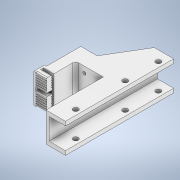
# Autodesk Inventor part: Soporte Linear Rail X
Saved by Autodesk Inventor 2021 (Build 250183000, 183)
## iProperties
Created: 2023-01-21
Part Number: Soporte Linear Rail X
Material: Plástico ABS
Document SubType Name: Modeling
Designer: Diego.labarca
Density: 1.06 g/cm^3
Appearance: Suave - Blanco
Author: Diego.labarca
Autodesk Inventor part; units mm, degrees
ref_plane "YZ Plane" through (0, 0, 0) normal (1, 0, 0) x (0, 1, 0)
ref_plane "XZ Plane" through (0, 0, 0) normal (0, 1, 0) x (-1, 0, 0)
ref_plane "XY Plane" through (0, 0, 0) normal (0, 0, 1) x (1, 0, 0)
sketch "Boceto1" plane through (0, 0, 0) normal (0, 0, 1) x (1, 0, 0)
  line L0 (-10, 11) -> (10, 11)
  line L1 (10, 11) -> (10, -11)
  line L2 (10, -11) -> (-10, -11)
  line L3 (-10, -11) -> (-10, 11)
  line L4 (1.6972, 0) -> (0, 0)
  line L5 (0, 0) -> (0, 1.3941)
  dimension "d11" = 22
  dimension "d12" = 20
  constraints: 12 end point, 2 horizontal, 2 parallel, 2 perpendicular, 2 other
  measures "d11" distance of L0.end L1.end
  measures "d12" distance of L0.start L0.end
extrude "Extrusión1" add sketch "Boceto1" along normal blind 15
sketch "Boceto5" plane through (0, 0, 15) normal (0, 0, 1) x (1, 0, 0)
  line L0 (-10, -11) -> (10, -11) projected
  line L1 (-10, -11) -> (35, -11)
  line L2 (35, -11) -> (35, -15)
  line L3 (35, -15) -> (-10, -15)
  line L4 (-10, -15) -> (-10, -11)
  line L5 (10, -11) -> (10, 11) projected
  line L6 (-10, 11) -> (-10, -11) projected
  line L7 (-10, 10) -> (35, 10)
  line L8 (35, 10) -> (35, 14)
  line L9 (35, 14) -> (-10, 14)
  line L10 (-10, 14) -> (-10, 10)
  line L11 (10, 11) -> (-10, 11) projected
  point P0 (0, 0)
  point P1 (10, 10)
  dimension "d25" = 4
  dimension "d26" = 25
  dimension "d28" = 4
  dimension "d29" = 1
  constraints: 16 end point, 4 parallel, 2 horizontal, 2 perpendicular, 1 collinear, 1 point on line
  measures "d25" distance of L1.end L2.end
  measures "d26" distance between parallel lines of L5 L2
  measures "d28" distance of L8.end L7.end
  measures "d29" distance from line of L7.start L11
extrude "Extrusión5" add sketch "Boceto5" against normal up to surface (15 mm away) contours L0 L1 L2 L3 L4 | L5 L11 L10 L9 L8 L7
sketch "Boceto7" plane through (0, 0, 0) normal (0, 0, -1) x (-1, 0, 0)
  line L0 (10, 14) -> (-35, 14) projected
  line L1 (-35, 10) -> (-10, 10) projected
  line L2 (-35, 14) -> (-15, 14)
  line L3 (-15, 14) -> (-15, 10)
  line L4 (-15, 10) -> (-35, 10)
  line L5 (-35, 10) -> (-35, 14)
  line L6 (-10, -11) -> (-35, -11) projected
  line L7 (-35, -15) -> (10, -15) projected
  line L8 (-35, -11) -> (-15, -11)
  line L9 (-15, -11) -> (-15, -15)
  line L10 (-15, -15) -> (-35, -15)
  line L11 (-35, -15) -> (-35, -11)
  point P0 (0, 0)
  point P1 (-15, 14)
  dimension "d32" = 20
  constraints: 16 end point, 4 parallel, 3 point on line, 2 horizontal, 2 perpendicular
  measures "d32" distance of L3.end L4.end
extrude "Extrusión6" add sketch "Boceto7" along normal blind 35 and the other way blind 71
ref_plane "Plano de trabajo1" through (0, 0, 7.5) normal (0, 0, -1) x (-1, 0, 0)
sketch "Boceto10" plane through (0, 0, -35) normal (0, 0, -1) x (-1, 0, 0)
  line L0 (10, 14) -> (-15, 14) projected
  line L1 (-10, 10) -> (-15, 10) projected
  line L2 (-15, 14) -> (-14, 14)
  line L3 (-14, 14) -> (-14, 10)
  line L4 (-14, 10) -> (-15, 10)
  line L5 (-15, 10) -> (-15, 14)
  line L6 (-15, -15) -> (-15, -11) projected
  line L7 (10, -15) -> (-15, -15) projected
  line L8 (-15, -11) -> (-14, -11)
  line L9 (-14, -11) -> (-14, -15)
  line L10 (-14, -15) -> (-15, -15)
  line L11 (-15, -15) -> (-15, -11)
  line L12 (-14, -15) -> (-11, -15)
  line L13 (-11, -15) -> (-11, 14)
  line L14 (-11, 14) -> (-14, 14)
  line L15 (-14, 14) -> (-14, -15)
  point P0 (0, 0)
  point P1 (-11, -15)
  point P2 (-11, 10)
  point P3 (-11, 14)
  dimension "d60" = 1
  dimension "d61" = 1
  dimension "d62" = 3
  constraints: 24 end point, 6 parallel, 3 horizontal, 3 perpendicular, 3 point on line
  measures "d60" distance of L3.end L4.end
  measures "d61" distance of L9.end L10.end
  measures "d62" distance of L14.end L13.end
extrude "Extrusión9" add sketch "Boceto10" against normal up to surface (106 mm away)
sketch "Boceto11" plane through (-10, 14, 15) normal (0, 1, 0) x (1, 0, 0)
  line L0 (0, 0) -> (0, 15) projected
  circle A0 centre (35, 7.5) radius 2.5
  circle A1 centre (35, 40) radius 2.5
  circle A2 centre (35, -41) radius 2.5
  line L1 (21, 50) -> (45, 50) projected
  line L2 (45, -56) -> (21, -56) projected
  line L3 (45, -56) -> (45, 50) projected
  point P0 (10, 15)
  dimension "d65" = 5
  dimension "d66" = 5
  dimension "d67" = 5
  dimension "d69" = 10
  dimension "d70" = 15
  dimension "d73" = 10
  dimension "d74" = 10
  dimension "d75" = 10
  constraints: 3 centre point
  measures "d65" diameter of A0
  measures "d66" diameter of A2
  measures "d67" diameter of A1
  measures "d69" distance from line of A1.centre L1
  measures "d70" distance from line of L2 A2.centre
  measures "d73" distance from line of L3 A2.centre
  measures "d74" distance from line of L3 A0.centre
  measures "d75" distance from line of L3 A1.centre
extrude "Extrusión10" cut sketch "Boceto11" against normal up to surface (29 mm away)
sketch "Boceto13" plane through (0, 0, 0) normal (0, 0, -1) x (-1, 0, 0)
  line L0 (-10, -11) -> (-10, 10) projected
  line L1 (-11, 10) -> (-10, 10) projected
  line L2 (-10, -11) -> (-11, -11) projected
  line L3 (-11, -15) -> (-11, 14) projected
  point P0 (0, 0)
extrude "Extrusión12" add sketch "Boceto13" against normal up to surface (15 mm away)
sketch "Boceto14" plane through (-10, 14, 15) normal (0, 1, 0) x (1, 0, 0)
  line L0 (21, 50) -> (45, 50) projected
  line L1 (0, 15) -> (21, 50)
  line L2 (21, 50) -> (21, 15) projected
  line L3 (0, 15) -> (21, 15) projected
  point P0 (10, 15)
  constraints: 2 end point
extrude "Extrusión13" add sketch "Boceto14" against normal up to surface (29 mm away)
sketch "Boceto12" plane through (11, -15, -35) normal (-1, 0, 0) x (0, 0, 1)
  circle A0 centre (15, 15) radius 2.5
  line L0 (0, 29) -> (35, 29) projected
  line L1 (0, 0) -> (0, 29) projected
  circle A1 centre (80, 15) radius 2.5
  line L2 (50, 29) -> (106, 29) projected
  line L3 (50, 29) -> (50, 0) projected
  line L4 (106, 0) -> (106, 29) projected
  point P0 (35, 15)
  dimension "d76" = 5
  dimension "d77" = 14
  dimension "d78" = 15
  dimension "d79" = 5
  dimension "d80" = 14
  dimension "d84" = 26
  constraints: 2 centre point
  measures "d76" diameter of A0
  measures "d77" distance from line of L0 A0.centre
  measures "d78" distance from line of L1 A0.centre
  measures "d79" diameter of A1
  measures "d80" distance from line of A1.centre L2
  measures "d84" distance from line of L4 A1.centre
extrude "Extrusión11" cut sketch "Boceto12" against normal through all both and the other way through all
sketch "Boceto15" plane through (-10, -15, 15) normal (-1, 0, 0) x (0, 0, 1)
  circle A0 centre (-35, 15) radius 2.5 projected
  circle A1 centre (-35, 15) radius 2.5 projected
  circle A2 centre (-35, 15) radius 5
  point P0 (-15, 15)
  dimension "d90" = 10
  constraints: 1 centre point, 1 coincident
  measures "d90" diameter of A2
extrude "Extrusión14" cut sketch "Boceto15" against normal blind 14 contours A0 | A2
sketch "Boceto16" plane through (0, 0, 15) normal (0, 0, 1) x (1, 0, 0)
  line L0 (2.28, 0) -> (0, 0)
  line L1 (0, 0) -> (0, 2.8237)
  circle A0 centre (7.5, 8) radius 1.5
  dimension "d93" = 8
  dimension "d94" = 7.5
  dimension "d113" = 3
  constraints: 4 end point, 1 centre point, 1 horizontal, 1 perpendicular
  measures "d93" distance from line of L0 A0.centre
  measures "d94" distance from line of L1 A0.centre
  measures "d113" diameter of A0
extrude "Extrusión15" cut sketch "Boceto16" against normal through all
pattern_linear "Patrón rectangular1" count 2 spacing 15 along (-1, 0, 0) count 2 spacing 16 along (0, -1, 0) of "Extrusión15"
ref_plane "Plano de trabajo2" through (0, 0, -2.5) normal (0, 0, 1) x (1, 0, 0)
sketch "Boceto17" plane through (0, 0, -2.5) normal (0, 0, 1) x (1, 0, 0)
  circle A0 centre (-7.5, 8) radius 1.5 projected
  circle A1 centre (-7.5, -8) radius 1.5 projected
  circle A2 centre (7.5, -8) radius 1.5 projected
  circle A3 centre (7.5, 8) radius 1.5 projected
  circle A4 centre (-7.5, 8) radius 3
  circle A5 centre (-7.5, -8) radius 3
  circle A6 centre (7.5, -8) radius 3
  circle A7 centre (7.5, 8) radius 3
  point P0 (0, 0)
  dimension "d104" = 6
  dimension "d105" = 6
  dimension "d106" = 6
  dimension "d107" = 6
  constraints: 4 centre point, 4 coincident
  measures "d104" diameter of A4
  measures "d105" diameter of A5
  measures "d106" diameter of A6
  measures "d107" diameter of A7
extrude "Extrusión16" cut sketch "Boceto17" against normal up to surface (32.5 mm away) contours A4 | A5
chamfer "Chaflán1" distance 1 angle 45 1 edges at (11, 0, 42.5)
ref_plane "Plano de trabajo3" through (0, 0, -12.5) normal (0, 0, 1) x (1, 0, 0)
sketch "Boceto18" plane through (0, 0, -12.5) normal (0, 0, 1) x (1, 0, 0)
  circle A0 centre (7.5, -8) radius 1.5 projected
  circle A1 centre (7.5, 8) radius 1.5 projected
  circle A2 centre (7.5, -8) radius 3
  circle A3 centre (7.5, 8) radius 3
  dimension "d115" = 6
  dimension "d116" = 6
  constraints: 2 centre point, 2 coincident
  measures "d115" diameter of A2
  measures "d116" diameter of A3
extrude "Extrusión17" cut sketch "Boceto18" against normal up to surface (22.5 mm away)
sketch "Boceto19" plane through (35, 14, 71) normal (0, 1, 0) x (1, 0, 0)
  line L0 (-24, 106) -> (0, 106) projected
  line L1 (0, 0) -> (-5, 0)
  line L2 (-5, 0) -> (-5, 106)
  line L3 (-5, 106) -> (0, 106)
  line L4 (0, 106) -> (0, 0)
  point P0 (-35, 71)
  dimension "d119" = 5
  constraints: 8 end point, 2 parallel, 1 horizontal, 1 perpendicular, 1 point on line
  measures "d119" distance of L2.end L3.end
extrude "Extrusión18" cut sketch "Boceto19" against normal up to surface (29 mm away)
sketch "Boceto20" plane through (-10, 14, 15) normal (0, 1, 0) x (1, 0, 0)
  line L0 (0, 0) -> (0, 15) projected
  line L1 (0, 15) -> (-6, 15)
  line L2 (-6, 15) -> (-6, 0)
  line L3 (-6, 0) -> (0, 0)
  line L4 (0, 0) -> (0, 15)
  line L5 (-6, 15) -> (-16, 15)
  line L6 (-16, 15) -> (-16, -29)
  line L7 (-16, -29) -> (-6, -29)
  line L8 (-6, -29) -> (-6, 15)
  point P0 (10, 15)
  point P1 (-6, 0)
  dimension "d122" = 10
  dimension "d123" = 44
  dimension "d124" = 6
  constraints: 16 end point, 4 parallel, 2 horizontal, 2 perpendicular
  measures "d122" distance of L7.end L6.end
  measures "d123" distance of L5.end L6.end
  measures "d124" distance of L0.end L1.end
extrude "Extrusión19" add sketch "Boceto20" against normal up to surface (29 mm away)
sketch "Boceto23" plane through (-26, 14, 0) normal (-1, 0, 0) x (0, 0, 1)
  line L0 (15, -29) -> (71, -29) projected
  line L1 (38, -29) -> (36.5, -29)
  line L2 (36.5, -29) -> (36.5, -14.5)
  line L3 (36.5, -14.5) -> (38, -14.5)
  line L4 (38, -14.5) -> (38, -29)
  line L5 (44, 0) -> (44, -29) projected
  line L6 (44, 0) -> (44, -29) projected
  line L7 (38, -14.5) -> (44, -14.5)
  line L8 (44, -14.5) -> (44, -16)
  line L9 (44, -16) -> (38, -16)
  line L10 (38, -16) -> (38, -14.5)
  point P0 (0, -14)
  point P1 (38, -16)
  point P2 (36.5, -29)
  dimension "d148" = 1.5
  dimension "d149" = 14.5
  dimension "d150" = 6
  dimension "d151" = 1.5
  constraints: 16 end point, 4 parallel, 2 horizontal, 2 perpendicular, 2 point on line
  measures "d148" distance of L2.end L3.end
  measures "d149" distance of L1.end L2.end
  measures "d150" distance between parallel lines of L5 L4
  measures "d151" distance between parallel lines of L9 L7
extrude "Extrusión22" cut sketch "Boceto23" against normal up to surface (10 mm away) contours L2 L3 L4 L0 | L4 L7 L5 L9
sketch "Boceto24" plane through (-26, -15, 38) normal (-1, 0, 0) x (0, 0, 1)
  line L0 (6, 13) -> (6, 0) projected
  line L1 (6, 0) -> (5.4, 0)
  line L2 (5.4, 0) -> (5.4, 1)
  line L3 (5.4, 1) -> (6, 1)
  line L4 (6, 1) -> (6, 0)
  point P0 (-38, 15)
  point P1 (6, 1)
  dimension "d154" = 0.6
  dimension "d155" = 1
  constraints: 8 end point, 2 parallel, 1 horizontal, 1 perpendicular
  measures "d154" distance of L2.end L3.end
  measures "d155" distance of L1.end L2.end
extrude "Extrusión23" cut sketch "Boceto24" against normal up to surface (10 mm away)
pattern_linear "Patrón rectangular3" count 6 spacing 2 along (0, 1, 0) count 2 spacing 5.4 along (0, 0, -1) of "Extrusión23"
sketch "Boceto25" plane through (-26, 14, 0) normal (-1, 0, 0) x (0, 0, 1)
  line L0 (44, 0) -> (44, -14.5) projected
  line L1 (0, -29) -> (36.5, -29) projected
  line L2 (15, -29) -> (71, -29) projected
  line L3 (44, -29) -> (33.5, -29)
  line L4 (33.5, -29) -> (33.5, -14.5)
  line L5 (33.5, -14.5) -> (44, -14.5)
  line L6 (44, -14.5) -> (44, -29)
  line L7 (36.5, -29) -> (36.5, -14.5) projected
  point P0 (0, -14)
  dimension "d165" = 14.5
  dimension "d166" = 3
  constraints: 8 end point, 2 parallel, 1 horizontal, 1 perpendicular, 1 point on line
  measures "d165" distance between parallel lines of L1 L5
  measures "d166" distance between parallel lines of L7 L4
extrude "Extrusión24" add sketch "Boceto25" along normal blind 2
mirror "Simetría3" about plane through (-26, -0.5, 44) normal (0, 1, 0) of "Extrusión22", "Extrusión23", "Patrón rectangular3", "Extrusión24"
fillet "Empalme3" radius 1 8 edges at (-21, -2, 44) (-21, -2, 38) (-21, -15, 43.4) (-21, -15, 38.6) (-21, 1, 44) (-21, 14, 38.6) (-21, 14, 43.4) (-21, 1, 38)
fillet "Empalme4" radius 3 1 edges at (-16, -0.5, 15)
equation "\"d25\" = d28"
equation "\"d66\" = d65"
equation "\"d67\" = d65"
equation "\"d74\" = d73"
equation "\"d75\" = d73"
equation "\"d79\" = d76"
equation "\"d80\" = d77"
equation "\"d105\" = d104"
equation "\"d106\" = d104"
equation "\"d107\" = d104"
equation "\"d151\" = d148"
